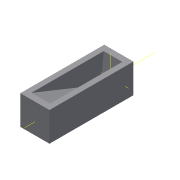
# Autodesk Inventor part: Mould Design
Saved by Autodesk Inventor 2015 (Build 190159000, 159)
## iProperties
Created: 2015-01-07
Part Number: Mould Design
Material: Generic
Document SubType Name: Modeling
Designer: I Rabey
Density: 1 g/cm^3
Appearance: Default
Author: I Rabey
Autodesk Inventor part; units mm, degrees
ref_plane "XZ Plane" through (0, 0, 0) normal (0, 1, 0) x (-1, 0, 0)
ref_plane "XY Plane" through (0, 0, 0) normal (0, 0, 1) x (1, 0, 0)
ref_plane "Work Plane1" through (8, 0, 0) normal (1, 0, 0) x (0, 1, 0)
sketch "Sketch4" plane through (8, 0, 0) normal (1, 0, 0) x (0, 1, 0)
  line L0 (-5, 0) -> (-5, 10)
  line L1 (15, 53) -> (15, -29) projected
  line L2 (-5, 0) -> (15, -2)
  line L3 (-5, 10) -> (15, 60)
  line L4 (15, 60) -> (15, -2)
  point P0 (0, 0)
  dimension "d9" = 10
  dimension "d10" = 20
  dimension "d11" = 2
  dimension "d12" = 60
  constraints: 8 end point, 2 point on line, 1 collinear, 1 vertical
  measures "d9" distance of L0.start L0.end
  measures "d10" distance from line of L1 L0.start
  measures "d11" vertical distance of point (0, 0) L2.end
  measures "d12" vertical distance of point (0, 0) L3.end
sketch "Sketch5" plane through (0, 0, 0) normal (0, 1, 0) x (-1, 0, 0)
  line L0 (12.5, 65) -> (-12.5, 65)
  line L1 (-12.5, 65) -> (-12.5, -7)
  line L2 (-12.5, -7) -> (12.5, -7)
  line L3 (12.5, -7) -> (12.5, 65)
  line L4 (12.5, 65) -> (-12.5, -7) construction
  line L5 (-12.5, 65) -> (12.5, -7) construction
  point P0 (0, 0)
  point P1 (0, 29)
  dimension "d13" = 25
  dimension "d14" = 72
  dimension "d15" = 7
  dimension "d22" = 0
  constraints: 12 end point, 2 midpoint, 2 parallel, 1 horizontal, 1 perpendicular
  measures "d13" distance of L2.end L1.end
  measures "d14" distance of L1.end L0.end
  measures "d15" distance from line of point (0, 0) L2
  measures "d22" horizontal distance of point (0, 0) point (0, 29)
extrude "Extrusion2" add sketch "Sketch5" along normal blind 15 and the other way blind 10
extrude "Extrusion3" cut sketch "Sketch4" against normal blind 16
body "Solid2"
